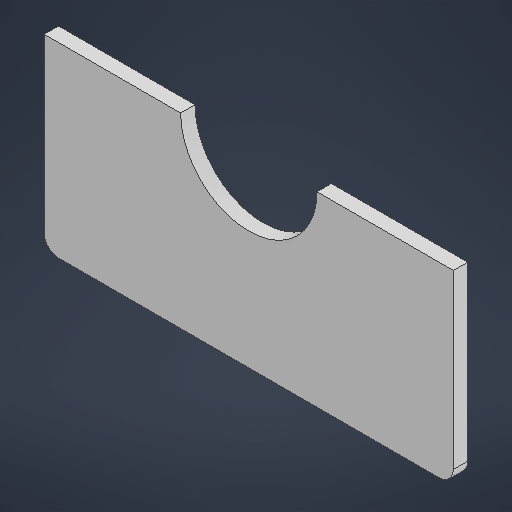
# Autodesk Inventor part: Bottom joint housing cover top back_ final
Saved by Autodesk Inventor 2026.3 (Build 303398000, 398)
## iProperties
Created: 2026-08-05
Part Number: Bottom joint housing cover top back_ final
Material: Generic
Document SubType Name: Sheet Metal
Designer: matot
Density: 1 g/cm^3
Sheet Metal Rule: Default_mm
Appearance: Default
Author: matot
Autodesk Inventor part; units mm, degrees
ref_plane "YZ Plane" through (0, 0, 0) normal (1, 0, 0) x (0, 1, 0)
ref_plane "XZ Plane" through (0, 0, 0) normal (0, 1, 0) x (-1, 0, 0)
ref_plane "XY Plane" through (0, 0, 0) normal (0, 0, 1) x (1, 0, 0)
sketch "Sketch1" plane through (0, 0, 0) normal (0, 0, 1) x (1, 0, 0)
  line L0 (-45, 30) -> (69, 30)
  line L1 (69, 30) -> (69, -18)
  line L2 (65, -22) -> (-41, -22)
  line L3 (-45, -18) -> (-45, 30)
  arc A0 (-45, -18) -> (-41, -22) centre (-41, -18) ccw
  arc A1 (65, -22) -> (69, -18) centre (65, -18) ccw
  point P0 (0, 0)
  dimension "d0" = 114
  dimension "d1" = 4
  dimension "d2" = 4
  dimension "d3" = 52
  measures "d0" distance of L0.start L0.end
  measures "d1" radius of A0
  measures "d2" radius of A1
  measures "d3" distance between parallel lines of L2 L0
extrude "Plate1" add sketch "Sketch1" along normal blind 4
sketch "Sketch2" plane through (0, 0, 4) normal (0, 0, 1) x (1, 0, 0)
  line L0 (69, 30) -> (-45, 30) projected
  arc A0 (-7, 30) -> (31, 30) centre (12, 30) ccw
  point P0 (0, 0)
  dimension "d5" = 38
  constraints: 2 point on circle, 2 point on line, 1 centre point, 1 midpoint
  measures "d5" diameter of A0
extrude "Extrusion1" cut sketch "Sketch2" against normal through all
equation "\"d4\" = Thickness"
equation "\"BendRadius\" = Thickness"
equation "\"BendReliefWidth\" = Thickness"
equation "\"BendReliefDepth\" = 0.5 * Thickness"
equation "\"CornerReliefSize\" = 4 * Thickness"
equation "\"MinimumRemnant\" = 2 * Thickness"
equation "\"TransitionRadius\" = BendRadius"
equation "\"JacobiRadiusSize\" = BendRadius"
equation "\"GapSize\" = Thickness"
equation "\"Thickness\" = 4"
body "Solid1"
